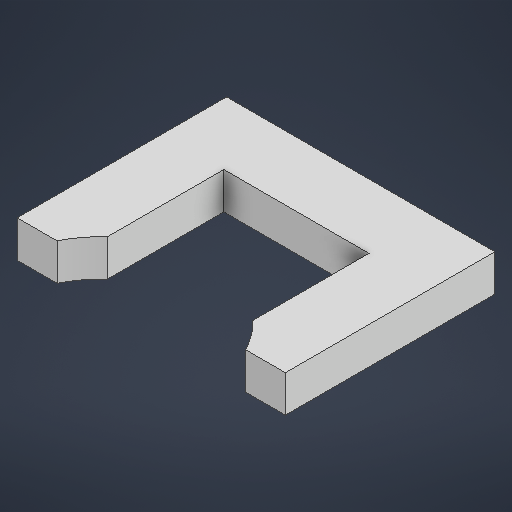
# Autodesk Inventor part: Spacer 1
Saved by Autodesk Inventor 2025 (Build 290162000, 162)
## iProperties
Created: 2024-06-12
Part Number: Spacer 1
Material: Generic
Document SubType Name: Modeling
Designer: mayhe
Density: 1 g/cm^3
Appearance: Default
Author: mayhe
Autodesk Inventor part; units mm, degrees
ref_plane "YZ Plane" through (0, 0, 0) normal (1, 0, 0) x (0, 1, 0)
ref_plane "XZ Plane" through (0, 0, 0) normal (0, 1, 0) x (-1, 0, 0)
ref_plane "XY Plane" through (0, 0, 0) normal (0, 0, 1) x (1, 0, 0)
sketch "Sketch1" plane through (0, 0, 0) normal (0, 1, 0) x (-1, 0, 0)
  line L0 (73, 70) -> (-73, 70)
  line L1 (-73, 70) -> (-73, -70)
  line L2 (-73, -70) -> (73, -70)
  line L3 (73, -70) -> (73, 70)
  line L4 (73, 70) -> (-73, -70) construction
  line L5 (-73, 70) -> (73, -70) construction
  line L6 (-73, -70) -> (73, -70)
  line L7 (73, -70) -> (73, 44)
  line L8 (73, 44) -> (-73, 44)
  line L9 (-73, 44) -> (-73, -70)
  circle A0 centre (0, 70) radius 57.5
  line L10 (39.5, 175) -> (-39.5, 175)
  line L11 (-39.5, 175) -> (-39.5, -35)
  line L12 (-39.5, -35) -> (39.5, -35)
  line L13 (39.5, -35) -> (39.5, 175)
  line L14 (39.5, 175) -> (-39.5, -35) construction
  line L15 (-39.5, 175) -> (39.5, -35) construction
  point P0 (0, 0)
  point P1 (-39.5, 28.2148)
  point P2 (-51.286, 44)
  point P3 (51.286, 44)
  point P4 (39.5, 28.2148)
  dimension "d0" = 146
  dimension "d1" = 140
  dimension "d2" = 114
  dimension "d3" = 115
  dimension "d4" = 210
  dimension "d5" = 79
  constraints: 32 end point, 6 parallel, 5 midpoint, 3 horizontal, 3 perpendicular, 1 centre point, 1 point on line
  measures "d0" distance of L2.end L1.end
  measures "d1" distance of L1.end L0.end
  measures "d2" distance of L7.end L6.end
  measures "d3" diameter of A0
  measures "d4" distance of L11.end L10.end
  measures "d5" distance of L11.end L12.end
extrude "Extrusion1" add sketch "Sketch1" along normal blind 20 contours L3 L2 L1 L8 A0 L11 L12 L13
sketch "Sketch2" plane through (0, 0, 0) normal (0, -1, 0) x (1, 0, 0)
  circle A0 centre (-43.5, -39) radius 2.75
  circle A1 centre (43.5, -39) radius 2.75
  line L0 (-39.5, 28.2148) -> (-39.5, -35) projected
  line L1 (-39.5, -35) -> (39.5, -35) projected
  line L2 (39.5, -35) -> (39.5, 28.2148) projected
  circle A2 centre (43.5, 6) radius 2.75
  circle A3 centre (-43.5, 6) radius 2.75
  point P0 (0, 0)
  dimension "d8" = 5.5
  dimension "d9" = 5.5
  dimension "d10" = 4
  dimension "d11" = 4
  dimension "d12" = 4
  dimension "d13" = 4
  dimension "d14" = 5.5
  dimension "d15" = 5.5
  dimension "d16" = 45
  dimension "d17" = 45
  constraints: 4 centre point, 2 vertical alignment
  measures "d8" diameter of A0
  measures "d9" diameter of A1
  measures "d10" distance from line of L0 A0.centre
  measures "d11" distance from line of L1 A0.centre
  measures "d12" distance from line of L1 A1.centre
  measures "d13" distance from line of L2 A1.centre
  measures "d14" diameter of A2
  measures "d15" diameter of A3
  measures "d16" distance of A1.centre A2.centre
  measures "d17" distance of A0.centre A3.centre
extrude "Extrusion2" cut sketch "Sketch2" against normal blind 2.5
body "Solid1"
